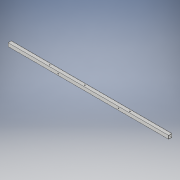
# Autodesk Inventor part: Lomg horizontal
Saved by Autodesk Inventor 2017 (Build 210142000, 142)
## iProperties
Created: 2018-07-12
Part Number: Lomg horizontal
Material: Generic
Document SubType Name: Modeling
Designer: sinner
Density: 1 g/cm^3
Appearance: Default
Author: sinner
Autodesk Inventor part; units mm, degrees
ref_plane "YZ Plane" through (0, 0, 0) normal (1, 0, 0) x (0, 1, 0)
ref_plane "XZ Plane" through (0, 0, 0) normal (0, 1, 0) x (-1, 0, 0)
ref_plane "XY Plane" through (0, 0, 0) normal (0, 0, 1) x (1, 0, 0)
sketch "Sketch1" plane through (0, 0, 0) normal (1, 0, 0) x (0, 1, 0)
  line L0 (0, 0) -> (25.4, 0)
  line L1 (25.4, 0) -> (25.4, -25.4)
  line L2 (25.4, -25.4) -> (0, -25.4)
  line L3 (0, -25.4) -> (0, 0)
  line L4 (23.8125, -23.8125) -> (23.8125, -1.5875)
  line L5 (23.8125, -1.5875) -> (1.5875, -1.5875)
  line L6 (1.5875, -1.5875) -> (1.5875, -23.8125)
  line L7 (1.5875, -23.8125) -> (23.8125, -23.8125)
  dimension "d0" = 25.4
  dimension "d1" = 25.4
  dimension "d2" = 1.5875
  constraints: 16 end point, 4 parallel, 2 perpendicular, 1 horizontal, 3 other
  measures "d0" distance of L1.end L2.end
  measures "d1" distance of L0.end L1.end
  measures "d2" distance between parallel lines of L1 L4
extrude "Extrusion1" add sketch "Sketch1" along normal blind 1219.2
sketch "Sketch3" plane through (0, 25.4, 0) normal (0, 1, 0) x (1, 0, 0)
  line L0 (0, 23.8125) -> (1219.2, 23.8125) projected
  line L1 (609.6, 23.8125) -> (609.6, 0) construction
  line L2 (0, 0) -> (1219.2, 0) projected
  line L3 (609.6, 11.9062) -> (465.3189, 11.9062) construction
  circle A0 centre (304.8, 11.9062) radius 3.175
  circle A1 centre (914.4, 11.9063) radius 3.175
  circle A2 centre (571.5, 11.9063) radius 3.175
  dimension "d10" = 6.35
  dimension "d11" = 304.8
  dimension "d14" = 38.1
  constraints: 4 end point, 3 centre point, 3 midpoint, 2 point on line, 1 equal radius, 1 horizontal, 1 symmetric about line, 1 other
  measures "d10" diameter of A0
  measures "d11" distance from line of L1 A0.centre
  measures "d14" distance from line of L1 A2.centre
extrude "Extrusion3" cut sketch "Sketch3" against normal blind 25.4
sketch "Sketch4" plane through (0, 0, 0) normal (0, 0, 1) x (1, 0, 0)
  line L0 (0, 0) -> (0, 25.4) projected
  line L1 (0, 12.7) -> (22.1319, 12.7) construction
  circle A0 centre (838.2, 12.7) radius 3.175
  line L2 (0, 0) -> (1219.2, 0) projected
  line L3 (609.6, 0) -> (609.6, 21.6417) construction
  circle A1 centre (381, 12.7) radius 3.175
  dimension "d15" = 6.35
  dimension "d19" = 228.6
  constraints: 4 end point, 2 centre point, 2 midpoint, 1 horizontal, 1 point on line, 1 symmetric about line, 1 vertical, 1 other
  measures "d15" diameter of A0
  measures "d19" distance from line of L3 A0.centre
extrude "Extrusion4" cut sketch "Sketch4" against normal blind 25.4
body "Solid1"
